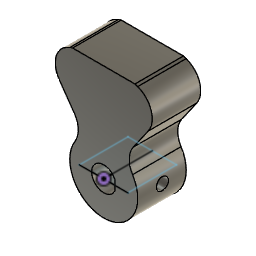
Turner Wiper (Autodesk Fusion 360 design; units mm, degrees)
Autodesk Fusion 360 part; units mm, degrees
note: some values were not read from the file. Chosen so that the rebuilt part matches the saved one: which face or edge a step refers to. Set by a fixed rule: which sketch regions a step uses.
sketch "Sketch1" plane through (0, 0, 0) normal (0, 1, 0) x (1, 0, 0)
  circle A0 centre (0, 0) radius 2.5
  circle A1 centre (0, 0) radius 21.15
  dimension "d1" = 5
  dimension "d2" = 42.3
  constraint coincident A0.centre A1.centre
  constraint concentric A0 A1
  measures "d1" diameter of A0
  measures "d2" diameter of A1
extrude "Extrude1" add sketch "Sketch1" along normal blind 10
ref_plane "WorkPlane1" through (0, 4.6027, 21.15) normal (0, 0, 1) x (-1, 0, 0)
sketch "Sketch2" plane through (0, 4.6027, 21.15) normal (0, 0, 1) x (1, 0, 0)
sketch "Sketch3" plane through (0, 0, 0) normal (0, 0, 1) x (1, 0, 0)
  line L0 (0, 0) -> (-5, 0)
  line L1 (-5, 0) -> (-5, 10)
  line L2 (-5, 10) -> (0, 10)
  line L3 (0, 10) -> (0, 0)
  line L4 (0, 0) -> (5, 0)
  line L5 (5, 0) -> (5, 10)
  line L6 (5, 10) -> (0, 10)
  line L7 (0, 10) -> (0, 0)
  constraint horizontal L0
  constraint vertical L1
  constraint horizontal L2
  constraint vertical L3
  constraint coincident L0.start L3.end
  constraint horizontal L4
  constraint vertical L5
  constraint horizontal L6
  constraint vertical L7
ref_plane "WorkPlane2" through (0, 0, 21.15) normal (0, 0, 1) x (1, 0, 0)
sketch "Sketch4" plane through (0, 0, 21.15) normal (0, 0, 1) x (1, 0, 0)
  line L0 (0, 0) -> (-5, 0)
  line L1 (-5, 0) -> (-5, 10)
  line L2 (-5, 10) -> (0, 10)
  line L3 (0, 10) -> (0, 0)
  line L4 (0, 0) -> (5, 0)
  line L5 (5, 0) -> (5, 10)
  line L6 (5, 10) -> (0, 10)
  line L7 (0, 10) -> (0, 0)
  constraint horizontal L0
  constraint vertical L1
  constraint horizontal L2
  constraint vertical L3
  constraint coincident L0.start L3.end
  constraint horizontal L4
  constraint vertical L5
  constraint horizontal L6
  constraint vertical L7
extrude "Extrude2" cut sketch "Sketch4" against normal blind 1
pattern_circular "C-Pattern1" count 2 over 360 about axis through (0, 10, 0) along (0, -1, 0) of "Extrude2"
sketch "Sketch5" plane through (0, 0, 0) normal (0, -1, 0) x (1, 0, 0)
  circle A0 centre (0, 0) radius 2.5
  line L0 (5, 20.15) -> (-5, 20.15)
  arc A1 (5, -20.5505) -> (5, 20.5505) centre (0, 0) ccw
  line L1 (-5, -20.15) -> (5, -20.15)
  line L2 (-5.104, 20.4487) -> (-5.4155, -20.3801) construction
  line L3 (5.104, 20.4487) -> (5.104, -20.4487) construction
  line L4 (5.4155, -20.3801) -> (20.3367, -10.7915) construction
  line L5 (0, 0) -> (5, 0)
  line L6 (5.4155, 20.3801) -> (20.3367, 10.7915) construction
  arc A2 (0, -8) -> (6.9282, -4) centre (0, 0) ccw
  arc A3 (0, -8) -> (0, -16) centre (0, -12) ccw
  arc A4 (0, -16) -> (13.8564, -8) centre (0, 0) ccw
  arc A5 (13.8564, -8) -> (6.9282, -4) centre (10.3923, -6) ccw
  arc A6 (0, -12) -> (10.3923, -6) centre (0, 0) ccw construction
  arc A7 (13.8564, 8) -> (0, 16) centre (0, 0) ccw
  arc A8 (6.9282, 4) -> (13.8564, 8) centre (10.3923, 6) ccw
  arc A9 (6.9282, 4) -> (0, 8) centre (0, 0) ccw
  arc A10 (0, 16) -> (0, 8) centre (0, 12) ccw
  arc A11 (-13.8564, 8) -> (-13.8564, -8) centre (0, 0) ccw
  arc A12 (-6.9282, 4) -> (-13.8564, 8) centre (-10.3923, 6) ccw
  arc A13 (-6.9282, 4) -> (-6.9282, -4) centre (0, 0) ccw
  arc A14 (-13.8564, -8) -> (-6.9282, -4) centre (-10.3923, -6) ccw
  line L7 (-5, 20.15) -> (-5, 20.5505)
  line L8 (5, 20.5505) -> (5, 20.15)
  arc A15 (-5, 20.5505) -> (-5, -20.5505) centre (0, 0) ccw
  line L9 (-5, -20.5505) -> (-5, -20.15)
  line L10 (5, -20.15) -> (5, -20.5505)
  dimension "d41" = 8
  dimension "d43" = 360
  constraint symmetric L4.start L5 L6.start
  constraint symmetric L4.end L5 L6.end
  constraint tangent A2 A3
  constraint tangent A3 A4
  constraint tangent A4 A5
  constraint tangent A2 A5
  constraint coincident A0.centre A1.centre
  measures "d41" diameter of A3
sketch "Sketch8" plane through (0, 0, -20.15) normal (0, 0, -1) x (1, 0, 0)
  line L0 (-5, -10) -> (5, -10)
  line L1 (5, 0) -> (-5, 0)
  line L2 (0, -10) -> (0, 0) construction
  line L3 (-4.7444, -5) -> (4.7444, -5) construction
  circle A0 centre (0, -5) radius 2.5
  line L4 (-5, 0) -> (-5, -10)
  line L5 (5, -10) -> (5, 0)
  dimension "d46" = 5
  constraint midpoint L0 L2.start
  constraint coincident L2.end origin
  constraint midpoint L2 A0.centre
  measures "d46" diameter of A0
ref_plane "WorkPlane3" through (4.1533, 6.45, -6.8374) normal (0.519167, 0, -0.854673) x (0.854673, 0, 0.519167)
sketch "Sketch9" plane through (4.1533, 6.45, -6.8374) normal (0.519167, 0, -0.854673) x (0.854673, 0, 0.519167)
  line L0 (0, -3.5) -> (0, 6.5) construction
  line L1 (0, -3.5) -> (0, 1.5) construction
  circle A0 centre (0, 1.5) radius 3
  dimension "d49" = 6
  constraint vertical L0
  constraint midpoint L0 L1.end
  constraint coincident L1.end A0.centre
  measures "d49" diameter of A0
sketch "Sketch11" plane through (3.8938, 0, -6.41) normal (0.519167, 0, -0.854673) x (0, 1, 0)
  circle A0 centre (4.95, 0) radius 3
sketch "Sketch12" plane through (3.8938, 0, -6.41) normal (0.519167, 0, -0.854673) x (0, 1, 0)
  circle A0 centre (4.95, 0) radius 1.6
  circle A1 centre (4.95, 0) radius 3
  dimension "d54" = 3.2
  measures "d54" diameter of A0
sketch "Sketch13" plane through (0, 10, 0) normal (0, 1, 0) x (-1, 0, 0)
  arc A0 (5, -20.5505) -> (5, 20.5505) centre (0, 0) ccw
  line L0 (-5, -20.15) -> (5, -20.15)
  line L1 (5, 20.15) -> (-5, 20.15)
  circle A1 centre (0, 0) radius 2.5
  circle A2 centre (0, 0) radius 7
  circle A3 centre (0, 0) radius 21.15
  line L2 (0, 0) -> (-12.1239, 17.3301)
  line L3 (0, 0) -> (0, 21.15) construction
  line L4 (0, 0) -> (12.1239, 17.3301)
  line L5 (0, 0) -> (21.15, 0.0085) construction
  line L6 (0, 0) -> (-12.11, -17.3399)
  line L7 (0, 0) -> (12.1379, -17.3204)
  line L8 (5, 20.5505) -> (5, 20.15)
  line L9 (-5, 20.15) -> (-5, 20.5505)
  line L10 (5, -20.15) -> (5, -20.5505)
  arc A4 (-5, 20.5505) -> (-5, -20.5505) centre (0, 0) ccw
  line L11 (-5, -20.5505) -> (-5, -20.15)
  dimension "d57" = 42.3
  constraint coincident A0.centre A1.centre
  constraint coincident A3 L2.end
  constraint coincident A0 L2.end
  constraint coincident A3 L3.end
  constraint perpendicular L1 L3
  constraint symmetric A0.centre L3 A1.centre
  constraint symmetric L2.end L3 L4.end
  constraint coincident A3 L5.end
  constraint symmetric A0.centre L5 A1.centre
  constraint symmetric L2.end L5 L6.end
  constraint symmetric L4.end L5 L7.end
  measures "d57" diameter of A3
extrude "Extrude6" cut sketch "Sketch13" against normal blind 12 contours L0 A3 L10 L11 | A0 A2 A3 L4 L7 | A2 A3 L2 L6 A4 | L1 A3 L8 L9
fillet "Fillet14" radius 4.5 2 edges at (-4.0126, 5, 5.7357) (-12.1239, 5, 17.3301)
fillet "Fillet15" radius 4.5 2 edges at (4.0126, 5, 5.7357) (12.1239, 5, 17.3301)
fillet "Fillet16" radius 4.5 4 edges at (4.008, 5, -5.739) (12.11, 5, -17.3399) (-4.0173, 5, -5.7325) (-12.1379, 5, -17.3204)
ref_plane "WorkPlane4" through (7, 5.1214, 0) normal (1, 0, 0) x (0, 0, -1)
sketch "Sketch17" plane through (0, 0, 0) normal (0, 1, 0) x (1, 0, 0)
  circle A0 centre (0, 0) radius 2.5
  line L0 (2.3, -0.9798) -> (2.3, 0.9798)
  dimension "d75" = 2.3
  constraint coincident A0.centre origin
  constraint coincident A0 L0.start
  constraint coincident A0 L0.end
  constraint vertical L0
  measures "d75" distance of A0.centre L0
extrude "Extrude10" add sketch "Sketch17" along normal blind 10 contours A0 L0 picked at (2.3368, -0.2211)
sketch "Sketch14" plane through (7, 5.1214, 0) normal (1, 0, 0) x (0, 1, 0)
  circle A0 centre (0, 0) radius 1.25
  circle A1 centre (0, 0) radius 2.9
  dimension "d67" = 2.5
  dimension "d70" = 5.8
  constraint coincident A0.centre A1.centre
  measures "d67" diameter of A0
  measures "d70" diameter of A1
extrude "Extrude7" cut sketch "Sketch14" against normal blind 5.5 contours A0
sketch "Sketch15" plane through (0, 0, 0) normal (0, -1, 0) x (1, 0, 0)
  arc A0 (-9.1997, -13.1277) -> (-7.005, -19.9563) centre (-5.5146, -15.7103) ccw
  arc A1 (-7.005, -19.9563) -> (-5, -20.5505) centre (0, 0) ccw
  line L0 (-5, -20.15) -> (5, -20.15)
  arc A2 (6.9729, -19.9675) -> (9.1786, -13.1425) centre (5.4893, -15.7191) ccw
  line L1 (9.1786, -13.1425) -> (6.0596, -8.6765)
  arc A3 (5.9341, -3.713) -> (6.0596, -8.6765) centre (9.7489, -6.0999) ccw
  arc A4 (5.9341, -3.713) -> (5.9371, 3.7082) centre (0, 0) ccw
  arc A5 (6.0666, 8.6716) -> (5.9371, 3.7082) centre (9.7538, 6.0921) ccw
  line L2 (6.0666, 8.6716) -> (9.1892, 13.1351)
  arc A6 (9.1892, 13.1351) -> (6.9889, 19.9619) centre (5.5019, 15.7147) ccw
  line L3 (5, 20.15) -> (-5, 20.15)
  arc A7 (-6.9889, 19.9619) -> (-9.1892, 13.1351) centre (-5.5019, 15.7147) ccw
  line L4 (-9.1892, 13.1351) -> (-6.0666, 8.6716)
  arc A8 (-5.9371, 3.7082) -> (-6.0666, 8.6716) centre (-9.7538, 6.0921) ccw
  arc A9 (-5.9371, 3.7082) -> (-5.9401, -3.7034) centre (0, 0) ccw
  arc A10 (-6.0735, -8.6667) -> (-5.9401, -3.7034) centre (-9.7587, -6.0842) ccw
  line L5 (-6.0735, -8.6667) -> (-9.1997, -13.1277)
  circle A11 centre (0, 0) radius 7
  line L6 (-5, 20.15) -> (-5, 20.5505)
  line L7 (5, 20.5505) -> (5, 20.15)
  line L8 (-5, -20.5505) -> (-5, -20.15)
  line L9 (5, -20.15) -> (5, -20.5505)
  arc A12 (5, -20.5505) -> (6.9729, -19.9675) centre (0, 0) ccw
  arc A13 (6.9889, 19.9619) -> (5, 20.5505) centre (0, 0) ccw
  arc A14 (-5, 20.5505) -> (-6.9889, 19.9619) centre (0, 0) ccw
  arc A15 (2.3, 0.9798) -> (2.3, -0.9798) centre (0, 0) ccw
  line L10 (2.3, 0.9798) -> (2.3, -0.9798)
  constraint concentric A1 A11
extrude "Extrude8" cut sketch "Sketch15" against normal blind 24 contours A0 A1 L0 A2 L1 A3 A10 L5 A11 L8 L9 A12
sketch "Sketch16" plane through (0, 0, 20.15) normal (0, 0, 1) x (-1, 0, 0)
  line L0 (5, 0) -> (-5, 0)
  line L1 (-5, 0) -> (-5, -10)
  line L2 (-5, -10) -> (5, -10)
  line L3 (5, -10) -> (5, 0)
  line L4 (14.8033, -13.3286) -> (-16.5048, -13.3286)
  line L5 (-16.5048, -13.3286) -> (-16.5048, 4.2255)
  line L6 (-16.5048, 4.2255) -> (14.8033, 4.2255)
  line L7 (14.8033, 4.2255) -> (14.8033, -13.3286)
  constraint horizontal L4
  constraint vertical L5
  constraint horizontal L6
  constraint vertical L7
extrude "Extrude9" cut sketch "Sketch16" along normal blind 5
